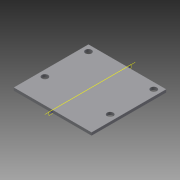
# Autodesk Inventor part: pcb
Saved by Autodesk Inventor 2014 (Build 180170000, 170)
## iProperties
Created: 2013-09-08
Part Number: pcb
Material: Generisch
Document SubType Name: Modeling
Designer: Felix
Density: 1 g/cm^3
Appearance: Vorgabe
Author: Felix
Autodesk Inventor part; units mm, degrees
ref_plane "YZ Plane" through (0, 0, 0) normal (1, 0, 0) x (0, 1, 0)
ref_plane "XZ Plane" through (0, 0, 0) normal (0, 1, 0) x (-1, 0, 0)
ref_plane "XY Plane" through (0, 0, 0) normal (0, 0, 1) x (1, 0, 0)
sketch "Skizze1" plane through (0, 0, 0) normal (0, 0, 1) x (1, 0, 0)
  line L0 (0, 0) -> (25, 0)
  line L1 (25, 0) -> (25, 24)
  line L2 (25, 24) -> (0, 24)
  line L3 (0, 24) -> (0, 0)
  circle A0 centre (2, 22) radius 1
  circle A1 centre (23, 22) radius 1
  circle A2 centre (2, 8) radius 1
  circle A3 centre (23, 8) radius 1
  dimension "d0" = 25
  dimension "d1" = 24
  dimension "d2" = 2
  dimension "d3" = 2
  dimension "d4" = 2
  dimension "d5" = 2
  dimension "d6" = 2
  dimension "d7" = 2
  dimension "d8" = 2
  dimension "d9" = 2
  dimension "d10" = 2
  dimension "d11" = 2
  dimension "d12" = 8
  dimension "d13" = 8
  constraints: 8 end point, 4 centre point, 2 parallel, 1 horizontal, 1 perpendicular
  measures "d0" distance of L2.end L1.end
  measures "d1" distance of L1.end L0.end
  measures "d2" diameter of A0
  measures "d3" diameter of A1
  measures "d4" diameter of A2
  measures "d5" diameter of A3
  measures "d6" distance from line of L2 A0.centre
  measures "d7" distance from line of L3 A0.centre
  measures "d8" distance from line of L1 A1.centre
  measures "d9" distance from line of A1.centre L2
  measures "d10" distance from line of L3 A2.centre
  measures "d11" distance from line of L1 A3.centre
  measures "d12" distance from line of A2.centre L0
  measures "d13" distance from line of L0 A3.centre
extrude "Extrusion1" add sketch "Skizze1" along normal blind 0.9
ref_plane "Arbeitsebene1" through (12.5, 24, 0.9) normal (-1, 0, 0) x (0, -1, 0)
